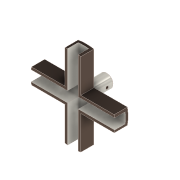
# Autodesk Inventor part: Cross
Saved by Autodesk Inventor 2022.2 (Build 262287010, 287A)
## iProperties
Created: 2022-12-29
Part Number: Cross
Material: Steel
Document SubType Name: Modeling
Designer: User
Mass: 58.03 g
Surface Area: 73.5155 cm^2
Volume: 7.39236 cm^3
Density: 7.85 g/cm^3
Appearance: Gunmetal - Antique Polished
Author: User
Autodesk Inventor part; units mm, degrees
ref_plane "YZ Plane" through (0, 0, 0) normal (1, 0, 0) x (0, 1, 0)
ref_plane "XY Plane" through (0, 0, 0) normal (0, 0, 1) x (1, 0, 0)
sketch "Sketch1" plane through (0, 0, 0) normal (0, 0, 1) x (1, 0, 0)
  circle A0 centre (0, 0) radius 32
  dimension "d0" = 64
  constraints: 1 centre point, 1 coincident
  measures "d0" diameter of A0
extrude "Extrusion1" add sketch "Sketch1" along normal blind 10
sketch "Sketch2" plane through (0, 0, 10) normal (0, 0, 1) x (1, 0, 0)
  circle A0 centre (0, 0) radius 32 projected
  line L0 (-31.4325, 6) -> (-6, 6)
  line L1 (-6, 6) -> (-6, 31.4325)
  dimension "d3" = 6
  constraints: 4 end point, 2 point on circle, 1 horizontal, 1 perpendicular, 1 vertical
  measures "d3" distance from line of A0.centre L1
extrude "Extrusion2" cut sketch "Sketch2" against normal through all contours L1 L0 A0 picked at (-8.4207, 22.185)
pattern_circular "Circular Pattern1" count 4 over 360 about axis through (0, 0, 0) along (0, 0, 1) of "Extrusion2"
sketch "Sketch3" plane through (0, 0, 10) normal (0, 0, 1) x (1, 0, 0)
  arc A0 (-31.4325, 6) -> (-31.4325, -6) centre (0, 0) ccw projected
  arc A1 (31.4325, -6) -> (31.4325, 6) centre (0, 0) ccw projected
  line L0 (-31.749, 4) -> (31.749, 4)
  line L1 (-31.749, -4) -> (31.749, -4)
  dimension "d9" = 8
  constraints: 4 end point, 4 point on circle, 2 horizontal, 1 parallel
  measures "d9" distance between parallel lines of L1 L0
extrude "Extrusion3" cut sketch "Sketch3" against normal blind 8
pattern_circular "Circular Pattern2" count 2 over 90 about axis through (0, 0, 0) along (0, 0, 1) of "Extrusion3"
sketch "Sketch4" plane through (0, 0, 0) normal (0, 0, -1) x (-1, 0, 0)
  arc A0 (6, 31.4325) -> (-6, 31.4325) centre (0, 0) ccw projected
  circle A1 centre (0, 0) radius 5
  dimension "d15" = 10
  constraints: 1 centre point, 1 coincident
  measures "d15" diameter of A1
extrude "Extrusion4" add sketch "Sketch4" along normal blind 16
chamfer "Chamfer1" distance 0.5 angle 45 1 edges at (5, 0, -16)
hole "Hole1" at (5, 0, -11) direction (-1, 0, 0) diameter 2 end through all
ref_plane "Work Plane1" through (0, 0, -11) normal (0, 0, -1) x (-1, 0, 0)
body "Solid1"
